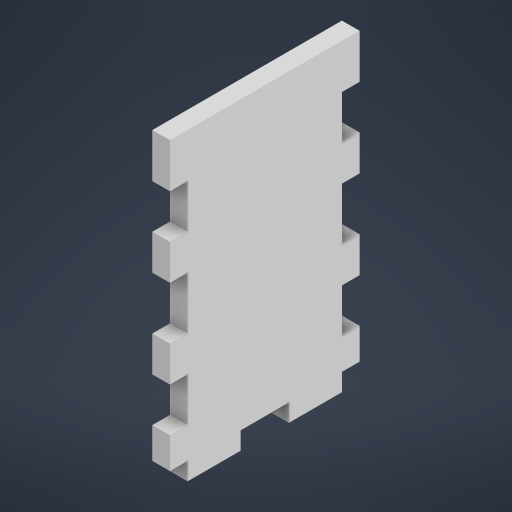
# Autodesk Inventor part: Langbektang houder
Saved by Autodesk Inventor 2023.2 (Build 272271000, 271)
## iProperties
Created: 2020-09-09
Part Number: Langbektang houder
Material: Generic
Document SubType Name: Modeling
Designer: nathan.bollaert
Density: 1 g/cm^3
Appearance: Default
Author: nathan.bollaert
Autodesk Inventor part; units mm, degrees
ref_plane "YZ Plane" through (0, 0, 0) normal (1, 0, 0) x (0, 1, 0)
ref_plane "XZ Plane" through (0, 0, 0) normal (0, 1, 0) x (-1, 0, 0)
ref_plane "XY Plane" through (0, 0, 0) normal (0, 0, 1) x (1, 0, 0)
sketch "Sketch1" plane through (0, 0, 0) normal (1, 0, 0) x (0, 1, 0)
  line L0 (0, 0) -> (69, 0)
  line L1 (69, 0) -> (69, -43)
  line L2 (69, -43) -> (0, -43)
  line L3 (0, -43) -> (0, 0)
  dimension "d228" = 69
  dimension "d229" = 43
  constraints: 8 end point, 2 parallel, 1 horizontal, 1 perpendicular
  measures "d228" distance of L1.end L2.end
  measures "d229" distance of L0.end L1.end
extrude "Extrusion1" add sketch "Sketch1" against normal blind 4
sketch "Sketch2" plane through (0, 0, 0) normal (1, 0, 0) x (0, 0, -1)
  line L0 (21.5, 69) -> (21.5, 0)
  line L1 (43, 0) -> (0, 0) projected
  line L2 (0, 0) -> (0, 69) projected
  line L3 (0, 34.5) -> (43, 34.5)
  line L4 (43, 69) -> (43, 0) projected
  line L5 (0, 0) -> (43, 0)
  line L6 (0, 4) -> (4, 4)
  line L7 (4, 4) -> (4, 0)
  line L8 (16, 0) -> (16, 4)
  line L9 (16, 4) -> (27, 4)
  line L10 (27, 4) -> (27, 0)
  line L11 (39, 0) -> (39, 4)
  line L12 (39, 4) -> (43, 4)
  line L13 (4, 0) -> (16, 0)
  line L14 (27, 0) -> (39, 0)
  line L15 (4, 59) -> (4, 49)
  line L16 (4, 49) -> (0, 49)
  line L17 (0, 49) -> (0, 41)
  line L18 (0, 41) -> (4, 41)
  line L19 (4, 41) -> (4, 29)
  line L20 (4, 29) -> (0, 29)
  line L21 (0, 29) -> (0, 21)
  line L22 (0, 21) -> (4, 21)
  line L23 (4, 21) -> (4, 11)
  line L24 (4, 11) -> (0, 11)
  line L25 (0, 69) -> (0, 0) projected
  line L26 (43, 0) -> (43, 69)
  line L27 (43, 34.5) -> (0, 34.5)
  line L28 (43, 49) -> (43, 41)
  line L29 (43, 29) -> (43, 21)
  line L30 (43, 69) -> (43, 0)
  line L31 (4, 59) -> (0, 59)
  line L32 (0, 0) -> (43, 0) projected
  line L33 (43, 69) -> (0, 69) projected
  line L34 (43, 0) -> (43, 69)
  line L35 (43, 34.5) -> (0, 34.5)
  line L36 (39, 59) -> (39, 49)
  line L37 (39, 49) -> (43, 49)
  line L38 (43, 49) -> (43, 41)
  line L39 (43, 41) -> (39, 41)
  line L40 (39, 41) -> (39, 29)
  line L41 (39, 29) -> (43, 29)
  line L42 (43, 29) -> (43, 21)
  line L43 (43, 21) -> (39, 21)
  line L44 (39, 21) -> (39, 11)
  line L45 (39, 11) -> (43, 11)
  line L46 (43, 69) -> (43, 0)
  line L47 (0, 34.5) -> (43, 34.5)
  line L48 (39, 59) -> (43, 59)
  point P0 (43, 65)
  point P1 (39, 0)
  point P2 (16, 0)
  point P3 (27, 0)
  point P4 (4, 0)
  dimension "d246" = 12
  dimension "d248" = 10
  dimension "d250" = 8
  dimension "d253" = 4
  dimension "d254" = 12
  dimension "d255" = 12
  dimension "d256" = 10
  constraints: 82 end point, 19 symmetric about line, 17 point on line, 11 equal length, 5 perpendicular, 3 horizontal, 2 midpoint, 1 vertical, 24 other
  measures "d246" distance of L17.end L20.end
  measures "d248" distance of L16.end L31.end
  measures "d250" distance of L16.end L17.end
  measures "d253" distance from line of L5 L6.start
  measures "d254" distance of L7.end L8.start
  measures "d255" distance of L11.start L10.end
  measures "d256" distance from line of L33 L31.end
extrude "Extrusion2" cut sketch "Sketch2" against normal blind 4 contours L9 L10 L1 L0 | L0 L1 L8 L9 | L19 L20 L2 L3 | L3 L2 L18 L19 | L40 L39 L4 L3 | L3 L4 L41 L40 | L4 L37 L36 L48 | L31 L15 L16 L2 | L11 L12 L4 L1 | L1 L2 L6 L7 | L22 L23 L24 L2 | L4 L45 L44 L43
body "Solid5"
